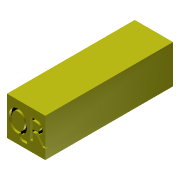
# Autodesk Inventor part: Container 2 2 5 QR color 6
Saved by Autodesk Inventor 2015 (Build 190159000, 159)
## iProperties
Created: 2015-03-07
Part Number: Container 2 2 5 QR color 6
Material: Generic
Document SubType Name: Modeling
Designer: Vukica
Density: 1 g/cm^3
Appearance: Yellow
Author: Vukica
Autodesk Inventor part; units mm, degrees
ref_plane "YZ Plane" through (0, 0, 0) normal (1, 0, 0) x (0, 1, 0)
ref_plane "XZ Plane" through (0, 0, 0) normal (0, 1, 0) x (-1, 0, 0)
ref_plane "XY Plane" through (0, 0, 0) normal (0, 0, 1) x (1, 0, 0)
sketch "Sketch1" plane through (0, 0, 0) normal (0, 0, 1) x (1, 0, 0)
  line L0 (0, 0) -> (38.1, 0)
  line L1 (38.1, 0) -> (38.1, 38.1)
  line L2 (38.1, 38.1) -> (0, 38.1)
  line L3 (0, 38.1) -> (0, 0)
  dimension "d0" = 38.1
  dimension "d1" = 38.1
  constraints: 8 end point, 2 parallel, 1 horizontal, 1 perpendicular
  measures "d0" distance of L1.end L2.end
  measures "d1" distance of L2.end L0.start
extrude "Extrusion1" add sketch "Sketch1" along normal blind 127
sketch "Sketch2" plane through (0, 0, 127) normal (0, 0, 1) x (1, 0, 0)
  line L0 (1.0317, 30.5311) -> (47.4268, 30.5311) construction
  line L1 (47.4268, 30.5311) -> (47.4268, -2.0937) construction
  line L2 (47.4268, -2.0937) -> (1.0317, -2.0937) construction
  line L3 (1.0317, -2.0937) -> (1.0317, 30.5311) construction
  spline S0 degree 2 poles (19.9684, 4.81) (19.2274, 4.6289) (17.6137, 4.4313) (16.8068, 4.4313) knots 0 0 0 1 2 2 2
  spline S1 degree 2 poles (16.8068, 4.4313) (14.5179, 4.4313) (11.6692, 6.9836) (11.5375, 9.3548) knots 0 0 0 1 2 2 2
  spline S2 degree 2 poles (11.5375, 9.3548) (11.3563, 9.3548) (11.0435, 9.3548) (10.9117, 9.3548) knots 0 0 0 1 2 2 2
  spline S3 degree 2 poles (10.9117, 9.3548) (8.8534, 9.3548) (5.5436, 10.7545) (4.3579, 12.1212) knots 0 0 0 1 2 2 2
  spline S4 degree 2 poles (4.3579, 12.1212) (3.1888, 13.4715) (1.9373, 17.4235) (1.9373, 19.9265) knots 0 0 0 1 2 2 2
  spline S5 degree 2 poles (1.9373, 19.9265) (1.9373, 22.4953) (3.2053, 26.3815) (4.3744, 27.7647) knots 0 0 0 1 2 2 2
  spline S6 degree 2 poles (4.3744, 27.7647) (5.56, 29.1314) (8.8698, 30.5311) (10.9117, 30.5311) knots 0 0 0 1 2 2 2
  spline S7 degree 2 poles (10.9117, 30.5311) (12.9865, 30.5311) (16.3128, 29.082) (17.4655, 27.7647) knots 0 0 0 1 2 2 2
  spline S8 degree 2 poles (17.4655, 27.7647) (18.6182, 26.4309) (19.9026, 22.4624) (19.9026, 19.9265) knots 0 0 0 1 2 2 2
  spline S9 degree 2 poles (19.9026, 19.9265) (19.9026, 15.9745) (16.8233, 10.8368) (14.1392, 9.9312) knots 0 0 0 1 2 2 2
  spline S10 degree 2 poles (14.1392, 9.9312) (14.2051, 9.1737) (14.6003, 7.9552) (14.9131, 7.6093) knots 0 0 0 1 2 2 2
  spline S11 degree 2 poles (14.9131, 7.6093) (15.2919, 7.1812) (16.3293, 6.786) (17.2514, 6.786) knots 0 0 0 1 2 2 2
  spline S12 degree 2 poles (17.2514, 6.786) (17.7948, 6.786) (19.2768, 7.1318) (19.6062, 7.2635) knots 0 0 0 1 2 2 2
  line L4 (19.6062, 7.2635) -> (19.9684, 7.2635)
  line L5 (19.9684, 7.2635) -> (19.9684, 4.81)
  spline S13 degree 2 poles (17.0868, 19.9265) (17.0868, 21.9519) (16.214, 25.0641) (15.4236, 26.0851) knots 0 0 0 1 2 2 2
  spline S14 degree 2 poles (15.4236, 26.0851) (14.6167, 27.1389) (12.3443, 28.1928) (10.9282, 28.1928) knots 0 0 0 1 2 2 2
  spline S15 degree 2 poles (10.9282, 28.1928) (9.4626, 28.1928) (7.2561, 27.1719) (6.4163, 26.0851) knots 0 0 0 1 2 2 2
  spline S16 degree 2 poles (6.4163, 26.0851) (5.6094, 25.0477) (4.7531, 21.9025) (4.7531, 19.9265) knots 0 0 0 1 2 2 2
  spline S17 degree 2 poles (4.7531, 19.9265) (4.7531, 15.9251) (8.1124, 11.6602) (10.9282, 11.6602) knots 0 0 0 1 2 2 2
  spline S18 degree 2 poles (10.9282, 11.6602) (13.744, 11.6602) (17.0868, 15.9251) (17.0868, 19.9265) knots 0 0 0 1 2 2 2
  line L6 (38.5924, 9.783) -> (35.0849, 9.783)
  line L7 (35.0849, 9.783) -> (28.6629, 17.8681)
  line L8 (28.6629, 17.8681) -> (25.5671, 17.8681)
  line L9 (25.5671, 17.8681) -> (25.5671, 9.783)
  line L10 (25.5671, 9.783) -> (22.8666, 9.783)
  line L11 (22.8666, 9.783) -> (22.8666, 30.103)
  line L12 (22.8666, 30.103) -> (28.103, 30.103)
  spline S19 degree 2 poles (28.103, 30.103) (29.8485, 30.103) (32.2033, 29.7242) (33.2736, 29.0326) knots 0 0 0 1 2 2 2
  spline S20 degree 2 poles (33.2736, 29.0326) (34.3439, 28.341) (35.5789, 26.1839) (35.5789, 24.5866) knots 0 0 0 1 2 2 2
  spline S21 degree 2 poles (35.5789, 24.5866) (35.5789, 22.3636) (33.3065, 19.3502) (31.3635, 18.6256) knots 0 0 0 1 2 2 2
  line L13 (31.3635, 18.6256) -> (38.5924, 9.783)
  spline S22 degree 2 poles (32.7631, 24.3725) (32.7631, 25.2617) (32.1374, 26.6285) (31.4787, 27.0731) knots 0 0 0 1 2 2 2
  spline S23 degree 2 poles (31.4787, 27.0731) (30.9024, 27.4518) (29.371, 27.7647) (28.2512, 27.7647) knots 0 0 0 1 2 2 2
  line L14 (28.2512, 27.7647) -> (25.5671, 27.7647)
  line L15 (25.5671, 27.7647) -> (25.5671, 20.1241)
  line L16 (25.5671, 20.1241) -> (27.9384, 20.1241)
  spline S24 degree 2 poles (27.9384, 20.1241) (29.1075, 20.1241) (30.9683, 20.5358) (31.6105, 21.178) knots 0 0 0 1 2 2 2
  spline S25 degree 2 poles (31.6105, 21.178) (32.2033, 21.7378) (32.7631, 23.3187) (32.7631, 24.3725) knots 0 0 0 1 2 2 2
  point P0 (0, 0)
  constraints: 2 other
extrude "Extrusion2" cut sketch "Sketch2" against normal blind 2.54
body "Solid1"
